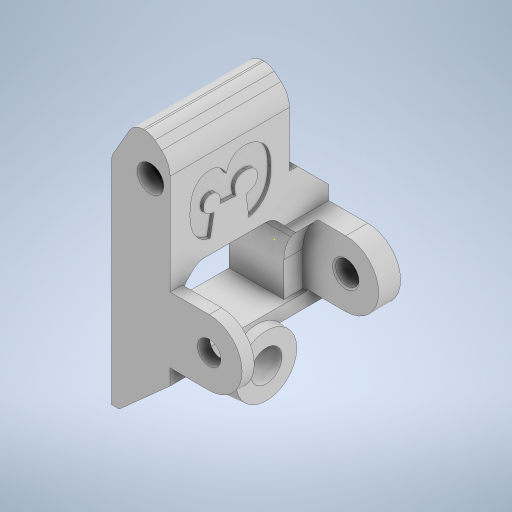
# Autodesk Inventor part: Extruder Idler V2
Saved by Autodesk Inventor 2023 (Build 270158000, 158)
## iProperties
Created: 2019-11-14
Part Number: Extruder Idler V2
Material: Generic
Document SubType Name: Modeling
Designer: pepd9
Density: 1 g/cm^3
Appearance: Default
Author: pepd9
Autodesk Inventor part; units mm, degrees
ref_plane "YZ Plane" through (0, 0, 0) normal (1, 0, 0) x (0, 1, 0)
ref_plane "XZ Plane" through (0, 0, 0) normal (0, 1, 0) x (-1, 0, 0)
ref_plane "XY Plane" through (0, 0, 0) normal (0, 0, 1) x (1, 0, 0)
sketch "Sketch1" plane through (0, 0, 0) normal (0, 0, 1) x (1, 0, 0)
  line L0 (-8.35, 16.25) -> (8.35, 16.25)
  line L1 (8.35, 16.25) -> (8.35, -16.25)
  line L2 (8.35, -16.25) -> (-8.35, -16.25)
  line L3 (-8.35, -16.25) -> (-8.35, 16.25)
  point P0 (0, 0)
  dimension "d2" = 16.7
  dimension "d3" = 8.35
  dimension "d4" = 32.5
  dimension "d5" = 16.25
  constraints: 8 end point, 2 parallel, 1 horizontal, 1 perpendicular
  measures "d2" distance of L0.start L0.end
  measures "d3" distance from line of L1 point (0, 0)
  measures "d4" distance of L0.end L1.end
  measures "d5" distance from line of point (0, 0) L0
extrude "Extrusion1" add sketch "Sketch1" along normal blind 25.5
sketch "Sketch3" plane through (0, 0, 0) normal (0, 0, -1) x (-1, 0, 0)
  line L0 (8.35, -16.25) -> (-8.35, -16.25) projected
  line L1 (8.35, 16.25) -> (8.35, -16.25) projected
  point P0 (0, 0)
  point P1 (-4.15, -4.25)
  dimension "d15" = 12
  dimension "d16" = 12.5
  measures "d15" distance from line of L0 point (-4.15, -4.25)
  measures "d16" distance from line of L1 point (-4.15, -4.25)
hole "Hole2" at (4.15, -4.25, 0) direction (0, 0, 1) diameter 2.99 end through all
sketch "Sketch4" plane through (0, 0, 0) normal (0, 0, -1) x (-1, 0, 0)
  line L0 (8.35, -16.25) -> (-8.35, -16.25) projected
  line L1 (-8.35, -16.25) -> (-8.35, 16.25) projected
  line L2 (8.35, 16.25) -> (8.35, -16.25) projected
  point P0 (0, 0)
  point P1 (3.35, 11.25)
  dimension "d24" = 27.5
  dimension "d36" = 5
  measures "d24" distance from line of L0 point (3.35, 11.25)
  measures "d36" distance from line of L2 point (3.35, 11.25)
hole "Hole3" at (-3.35, 11.25, 0) direction (0, 0, 1) diameter 3.4 end through all
sketch "Sketch5" plane through (0, 0, 0) normal (0, 0, -1) x (-1, 0, 0)
  circle A0 centre (3.35, 11.25) radius 1.7 projected
  line L0 (-8.35, 16.25) -> (8.35, 16.25) projected
  line L1 (8.35, 16.25) -> (8.35, -16.25) projected
  line L2 (-8.35, 16.25) -> (8.35, 16.25)
  line L3 (8.35, 16.25) -> (8.35, 5.75)
  line L4 (8.35, 5.75) -> (-8.35, 5.75)
  line L5 (-8.35, 5.75) -> (-8.35, 16.25)
  point P0 (0, 0)
  dimension "d33" = 5.5
  constraints: 8 end point, 2 parallel, 1 horizontal, 1 perpendicular, 1 point on line
  measures "d33" distance from line of L4 A0.centre
extrude "Extrusion2" cut sketch "Sketch5" against normal blind 5
sketch "Sketch6" plane through (0, 0, 0) normal (0, 0, -1) x (-1, 0, 0)
  line L0 (8.35, 5.75) -> (-8.35, 5.75) projected
  line L1 (-8.35, -16.25) -> (-8.35, 5.75) projected
  line L2 (8.35, -16.25) -> (-8.35, -16.25) projected
  line L3 (8.35, 5.75) -> (8.35, -16.25) projected
  circle A0 centre (-4.15, -4.25) radius 1.495 projected
  circle A1 centre (-4.15, -4.25) radius 4.2
  line L4 (-8.35, -16.25) -> (-8.35, 5.75) projected
  line L5 (-8.35, 5.75) -> (-8.35, 16.25) projected
  line L6 (8.35, 5.75) -> (-8.35, 5.75) projected
  line L7 (8.35, 16.25) -> (8.35, 5.75) projected
  line L8 (-8.35, 16.25) -> (8.35, 16.25) projected
  circle A2 centre (3.35, 11.25) radius 1.7 projected
  line L9 (-4.15, -0.05) -> (-2.65, -0.05)
  line L10 (-2.65, -0.05) -> (-2.65, 0.45)
  line L11 (-2.65, 0.45) -> (0.35, 16.25)
  line L12 (-8.35, 16.25) -> (8.35, 16.25) projected
  point P0 (0, 0)
  point P1 (0.35, 16.25)
  point P2 (-8.35, -4.25)
  dimension "d37" = 1.5
  dimension "d38" = 0.5
  dimension "d39" = 3
  constraints: 6 end point, 2 horizontal, 2 vertical, 1 coincident, 1 point on line, 3 other
  measures "d37" distance of L9.end L9.start
  measures "d38" distance of L9.end L10.end
  measures "d39" horizontal distance of A2.centre L11.end
extrude "Extrusion3" cut sketch "Sketch6" against normal through all contours L11 L10 L9 A1 L1 L0 | L0 L5 L8 L11
chamfer "Chamfer1" distance 3 angle 45 1 edges at (-0.35, 16.25, 15.25)
chamfer "Chamfer2" distance 5 angle 30 1 edges at (-8.35, 16.25, 15.25) measured on face at (-8.35, 15.75, 15.25)
ref_plane "Work Plane1" through (0, 0, 3.8) normal (0, 0, -1) x (-1, 0, 0)
sketch "Sketch7" plane through (0, 0, 3.8) normal (0, 0, -1) x (-1, 0, 0)
  arc A0 (-4.15, -0.05) -> (-8.35, -4.25) centre (-4.15, -4.25) ccw projected
  line L0 (-8.35, -16.25) -> (-8.35, -4.25) projected
  line L1 (8.35, -16.25) -> (-8.35, -16.25) projected
  line L2 (8.35, 5.75) -> (8.35, -16.25) projected
  line L3 (8.35, 5.75) -> (-1.6437, 5.75) projected
  line L4 (-1.6437, 5.75) -> (-2.65, 0.45) projected
  line L5 (-2.65, 0.45) -> (-2.65, -0.05) projected
  line L6 (-2.65, -0.05) -> (-4.15, -0.05) projected
  circle A1 centre (-4.15, -4.25) radius 1.495 projected
  circle A2 centre (-4.15, -4.25) radius 1.495 projected
  circle A3 centre (-4.15, -4.25) radius 5.5
  line L7 (1.35, -4.25) -> (-4.15, -4.25)
  line L8 (-4.15, -4.25) -> (-4.15, -9.75)
  line L9 (-4.15, -9.75) -> (1.35, -9.75)
  line L10 (1.35, -9.75) -> (1.35, -4.25)
  point P0 (0, 0)
  dimension "d49" = 11
  constraints: 8 end point, 2 parallel, 2 point on circle, 1 centre point, 1 coincident, 1 horizontal, 1 perpendicular
  measures "d49" diameter of A3
extrude "Extrusion4" cut sketch "Sketch7" against normal blind 5 contours L6 L5 L4 A3 L7 A1 L8 L0 A0 | A0 L0 A3 L4 L5 L6 | L8 A1 L7 A3 | A3 L10 L9 | L8 L7 A1 | A1 L7 L8
sketch "Sketch8" plane through (0, 0, 8.8) normal (0, 0, -1) x (-1, 0, 0)
  point P0 (0, 0)
sketch "Sketch9" plane through (0, 0, 8.8) normal (0, 0, -1) x (-1, 0, 0)
  circle A0 centre (-4.15, -4.25) radius 1.495 projected
  circle A1 centre (-4.15, -4.25) radius 5
  line L0 (-2.65, 0.45) -> (-2.5436, 1.0102) projected
  line L1 (-2.65, -0.05) -> (-2.65, 0.45) projected
  line L2 (-4.15, -0.05) -> (-2.65, -0.05) projected
  arc A2 (-4.15, -0.05) -> (-8.35, -4.25) centre (-4.15, -4.25) ccw projected
  line L3 (-8.35, -7.8011) -> (-8.35, -4.25) projected
  arc A3 (-8.35, -7.8011) -> (-4.15, -9.75) centre (-4.15, -4.25) ccw projected
  line L4 (1.35, -9.75) -> (-4.15, -9.75) projected
  line L5 (1.35, -4.25) -> (1.35, -9.75) projected
  arc A4 (1.35, -4.25) -> (-2.5436, 1.0102) centre (-4.15, -4.25) ccw projected
  circle A5 centre (-4.15, -4.25) radius 1.495 projected
  line L6 (-4.15, -9.25) -> (-9.15, -9.25)
  line L7 (-9.15, -9.25) -> (-9.15, -4.25)
  line L8 (-9.15, -4.25) -> (-4.15, -4.25)
  line L9 (-4.15, -4.25) -> (-4.15, -9.25)
  point P0 (0, 0)
  dimension "d52" = 10
  constraints: 8 end point, 2 parallel, 2 point on circle, 1 centre point, 1 coincident, 1 horizontal, 1 perpendicular
  measures "d52" diameter of A1
extrude "Extrusion5" cut sketch "Sketch9" against normal blind 9.4 contours A0 L8 A2 L2 L1 L0 A1 L9 | A0 L9 A1 L3 L8 | L8 A1 L0 L1 L2 A2 | L3 A1 L8 | L6 A3 L3 A1 | L3 A3 L6 L7 A1
ref_plane "Work Plane2" through (0, 0, 22) normal (0, 0, -1) x (-1, 0, 0)
sketch "Sketch10" plane through (0, 0, 22) normal (0, 0, -1) x (-1, 0, 0)
  circle A0 centre (-4.15, -4.25) radius 1.495 projected
  line L0 (-8.35, -9.25) -> (-8.35, -4.25) projected
  arc A1 (-4.15, -9.25) -> (-2.6375, 0.5158) centre (-4.15, -4.25) ccw projected
  line L1 (-2.65, 0.45) -> (-2.6375, 0.5158) projected
  line L2 (-2.65, -0.05) -> (-2.65, 0.45) projected
  line L3 (-4.15, -0.05) -> (-2.65, -0.05) projected
  arc A2 (-4.15, -0.05) -> (-8.35, -4.25) centre (-4.15, -4.25) ccw projected
  line L4 (-4.15, -9.25) -> (-8.35, -9.25) projected
  point P0 (0, 0)
extrude "Extrusion6" cut sketch "Sketch10" against normal through all
sketch "Sketch11" plane through (0, 0, 0) normal (0, 0, -1) x (-1, 0, 0)
  circle A0 centre (-4.15, -4.25) radius 1.495 projected
  line L0 (-1.6437, 5.75) -> (-2.65, 0.45) projected
  line L1 (-2.65, 0.45) -> (-2.65, -0.05) projected
  line L2 (-2.65, -0.05) -> (-4.15, -0.05) projected
  arc A1 (-4.15, -0.05) -> (-8.35, -4.25) centre (-4.15, -4.25) ccw projected
  line L3 (-8.35, -16.25) -> (-8.35, -4.25) projected
  line L4 (8.35, -16.25) -> (-8.35, -16.25) projected
  line L5 (8.35, 5.75) -> (8.35, -16.25) projected
  line L6 (8.35, 5.75) -> (-1.6437, 5.75) projected
  arc A2 (-4.15, -0.05) -> (-8.35, -4.25) centre (-4.15, -4.25) ccw projected
  circle A3 centre (-4.15, -4.25) radius 4.2
  line L7 (-4.15, -8.45) -> (0.85, -8.45)
  line L8 (8.35, -16.25) -> (-8.35, -16.25) projected
  line L9 (8.35, -16.25) -> (7.35, -16.25)
  line L10 (0.85, -8.45) -> (0.85, -10.45)
  line L11 (0.85, -10.45) -> (7.35, -16.25)
  point P0 (0, 0)
  dimension "d58" = 1
  dimension "d59" = 5
  dimension "d60" = 2
  constraints: 8 end point, 2 point on circle, 1 centre point, 1 coincident, 1 collinear, 1 horizontal, 1 point on line, 1 vertical
  measures "d58" distance of L4.start L9.end
  measures "d59" distance of L7.start L7.end
  measures "d60" distance of L7.end L10.end
extrude "Extrusion7" cut sketch "Sketch11" against normal through all contours L4 L3 A3 L7 L10 L11
fillet "Fillet1" radius 2 1 edges at (1.4371, -8.45, 23.75)
chamfer "Chamfer3" distance 0.2 angle 45 4 edges at (4.15, -5.745, 0) (4.15, -5.745, 18.2) (4.15, -5.745, 3.8) (4.15, -5.745, 22)
fillet "Fillet3" radius 2 4 edges at (0.2096, 13.3027, 15.25) (-3.35, 16.25, 15.25) (-5.4632, 16.25, 15.25) (-8.35, 11.25, 15.25)
sketch "Sketch12" plane through (-8.35, 5.75, 0) normal (-1, 0, 0) x (0, 0, 1)
  line L0 (18.1, -6.1) -> (18.1, -13.9) projected
  line L1 (3.8, -11.695) -> (3.8, -8.305) projected
  line L2 (3.8, -5.3) -> (3.8, -5.8) projected
  line L3 (3.8, -4.7398) -> (3.8, -5.3) projected
  line L4 (3.8, -10) -> (3.8, -4.7398) projected
  line L5 (3.8, -15.5) -> (3.8, -10) projected
  line L6 (18.2, -14.2) -> (18.2, -5.2342) projected
  line L7 (18.2, -14.2) -> (6.2, -14.2)
  line L8 (6.2, -14.2) -> (6.2, -4.2)
  line L9 (6.2, -4.2) -> (18.2, -4.2)
  line L10 (18.2, -4.2) -> (18.2, -14.2)
  line L11 (6.2, -14.2) -> (18.2, -14.2)
  line L12 (18.2, -14.2) -> (18.2, -16.2)
  line L13 (18.2, -16.2) -> (6.2, -16.2)
  line L14 (6.2, -16.2) -> (6.2, -14.2)
  line L15 (3.8, -15.5) -> (3.8, -14.2) projected
  line L16 (3.8, -14.2) -> (3.8, -5.8) projected
  point P0 (0, -5.75)
  dimension "d88" = 12
  dimension "d89" = 10
  dimension "d90" = 2
  constraints: 16 end point, 4 parallel, 2 horizontal, 2 perpendicular, 1 vertical alignment
  measures "d88" distance of L8.end L9.end
  measures "d89" distance of L7.end L8.end
  measures "d90" distance of L11.end L12.end
extrude "Extrusion8" cut sketch "Sketch12" against normal through all
sketch "Sketch13" plane through (-8.35, 5.75, 0) normal (-1, 0, 0) x (0, 0, 1)
  line L0 (5, 9.5) -> (5, 5.9641) projected
  line L1 (25.5, 5.9641) -> (25.5, 9.5) projected
  circle A0 centre (15.4, 10.3352) radius 2
  line L2 (15.4, 10.3352) -> (15.4, -24.7927)
  circle A1 centre (10.1533, -18.9) radius 4.5
  line L3 (18.1, -13.9) -> (5.8, -13.9) projected
  point P0 (0, -5.75)
  dimension "d81" = 4
  dimension "d82" = 9
  dimension "d83" = 5
  constraints: 2 centre point, 2 coincident, 2 end point, 1 vertical, 1 other
  measures "d81" diameter of A0
  measures "d82" diameter of A1
  measures "d83" distance from line of L3 point (10.153, -18.9)
extrude "Extrusion9" add sketch "Sketch13" against normal blind 8.7 contours A1
chamfer "Chamfer5" distance 2 angle 45 2 edges at (-2.9544, 1.55, 6.2) (-2.9544, 1.55, 18.2)
sketch "Sketch14" plane through (-8.35, 5.75, 0) normal (-1, 0, 0) x (0, 0, 1)
  arc A0 (6.8914, -22) -> (13.4152, -22) centre (10.1533, -18.9) ccw projected
  point P0 (0, -5.75)
hole "Hole4" at (-8.35, -13.15, 10.1533) direction (1, 0, 0) diameter 4 end through all counterbore diameter 7.4 counterbore depth 5
fillet "Fillet4" radius 2 2 edges at (-7.85, -16.25, 13.4152) (-7.85, -16.25, 6.8914)
fillet "Fillet5" radius 2 4 edges at (-1.2056, -0.45, 18.2) (-2.9544, 1.55, 16.2) (-2.9544, 1.55, 8.2) (-4.0881, -0.45, 6.2)
sketch "Sketch15" plane through (-8.35, -10.45, 6.2) normal (0, 0, 1) x (1, 0, 0)
  line L0 (0, 9.1716) -> (7.8719, 9.1716) projected
  line L1 (0, 0) -> (0, 9.1716) projected
  line L2 (0, 0) -> (7.5, 0) projected
  line L3 (7.5, 0.7) -> (7.5, 0) projected
  line L4 (7, 0.7) -> (7.5, 0.7) projected
  line L5 (7, 6.2) -> (7, 0.7) projected
  arc A0 (7.8719, 9.1716) -> (7, 6.2) centre (12.5, 6.2) ccw projected
  line L6 (0, 1.8) -> (8.7, 1.8) projected
  point P0 (8.35, 10.45)
  point P1 (7, 1.8)
extrude "Extrusion10" add sketch "Sketch15" along normal up to surface contours L6 L5 L4 L3 L2 L1 round surface about axis through (-8.35, -13.15, 10.1533) along (1, 0, 0) radius 4.5 far side no
sketch "Sketch16" plane through (0, 0, 18.2) normal (0, 0, -1) x (-1, 0, 0)
  line L0 (8.35, -8.65) -> (1.35, -8.65) projected
  line L1 (-7.1181, -1.2784) -> (8.35, -1.2784) projected
  arc A0 (-7.1181, -1.2784) -> (-4.15, -8.45) centre (-4.15, -4.25) ccw projected
  line L2 (-4.15, -8.45) -> (0.85, -8.45) projected
  line L3 (0.85, -10.45) -> (0.85, -8.45) projected
  line L4 (8.35, -10.45) -> (0.85, -10.45) projected
  line L5 (8.35, -1.2784) -> (8.35, -10.45) projected
  circle A1 centre (-4.15, -4.25) radius 1.695 projected
  line L6 (1.35, -8.65) -> (0.85, -8.65)
  line L7 (0.85, -10.45) -> (0.85, -8.45) projected
  point P0 (0, 0)
  constraints: 2 end point, 1 perpendicular, 1 point on line
extrude "Extrusion11" add sketch "Sketch16" along normal up to surface contours L5 L4 L3 L6 L0 round surface about axis through (-8.35, -13.15, 10.1533) along (1, 0, 0) radius 4.5 far side no
sketch "Sketch17" plane through (0, 0, 3.8) normal (0, 0, 1) x (1, 0, 0)
  arc A0 (-8.0821, 11.7141) -> (-8.35, 10.7141) centre (-6.35, 10.7141) ccw projected
  line L0 (-8.35, 10.7141) -> (-8.35, -16.25) projected
  line L1 (-8.35, -16.25) -> (-7.35, -16.25) projected
  line L2 (-7.35, -16.25) -> (-0.85, -10.45) projected
  line L3 (-0.85, -10.45) -> (-0.85, -8.45) projected
  arc A1 (-0.85, -8.45) -> (-0.4353, -6.2436) centre (-2.2695, -7.0411) ccw projected
  arc A2 (2.6375, 0.5158) -> (-0.4353, -6.2436) centre (4.15, -4.25) ccw projected
  line L4 (2.6375, 0.5158) -> (0.344, 12.5948) projected
  arc A3 (0.344, 12.5948) -> (-0.3454, 13.7622) centre (-1.6209, 12.2217) ccw projected
  line L5 (-2.795, 15.7905) -> (-0.3454, 13.7622) projected
  arc A4 (-2.795, 15.7905) -> (-4.0705, 16.25) centre (-4.0705, 14.25) ccw projected
  line L6 (-4.0705, 16.25) -> (-4.3085, 16.25) projected
  arc A5 (-4.3085, 16.25) -> (-6.0406, 15.25) centre (-4.3085, 14.25) ccw projected
  line L7 (-8.0821, 11.7141) -> (-6.0406, 15.25) projected
  circle A6 centre (-3.35, 11.25) radius 1.7 projected
  line L8 (-0.85, -9.75) -> (-0.85, -8.45) projected
  line L9 (-0.85, -8.45) -> (4.15, -8.45) projected
  arc A7 (4.15, -8.45) -> (4.15, -0.05) centre (4.15, -4.25) ccw projected
  line L10 (2.65, -0.05) -> (4.15, -0.05) projected
  line L11 (2.65, 0.45) -> (2.65, -0.05) projected
  line L12 (2.5436, 1.0102) -> (2.65, 0.45) projected
  arc A8 (2.5436, 1.0102) -> (-1.35, -4.25) centre (4.15, -4.25) ccw projected
  line L13 (-1.35, -9.75) -> (-1.35, -4.25) projected
  line L14 (-0.85, -9.75) -> (-1.35, -9.75) projected
  circle A9 centre (4.15, -4.25) radius 1.695 projected
  line L15 (-0.85, -8.45) -> (-1.35, -8.45)
  line L16 (-0.85, -8.65) -> (-1.35, -8.65) projected
  point P0 (0, 0)
  constraints: 2 end point, 1 horizontal, 1 point on line
extrude "Extrusion12" add sketch "Sketch17" along normal up to surface contours L14 L13 L16 L3 round surface about axis through (-8.35, -13.15, 10.1533) along (1, 0, 0) radius 4.5 far side no
chamfer "Chamfer6" distance 7 angle 5 1 edges at (0.35, -13.15, 5.6533) measured on face at (-0.15, -13.15, 5.6533)
sketch "Sketch18" plane through (0, 0, 25.5) normal (0, 0, 1) x (1, 0, 0)
  arc A0 (-8.0821, 11.7141) -> (-8.35, 10.7141) centre (-6.35, 10.7141) ccw projected
  line L0 (-8.35, 10.7141) -> (-8.35, -16.25) projected
  line L1 (-8.35, -16.25) -> (-7.35, -16.25) projected
  line L2 (-7.35, -16.25) -> (-0.85, -10.45) projected
  line L3 (-0.85, -10.45) -> (-0.85, -8.45) projected
  arc A1 (-0.85, -8.45) -> (-0.4353, -6.2436) centre (-2.2695, -7.0411) ccw projected
  arc A2 (2.6375, 0.5158) -> (-0.4353, -6.2436) centre (4.15, -4.25) ccw projected
  line L4 (2.6375, 0.5158) -> (0.344, 12.5948) projected
  arc A3 (0.344, 12.5948) -> (-0.3454, 13.7622) centre (-1.6209, 12.2217) ccw projected
  line L5 (-2.795, 15.7905) -> (-0.3454, 13.7622) projected
  arc A4 (-2.795, 15.7905) -> (-4.0705, 16.25) centre (-4.0705, 14.25) ccw projected
  line L6 (-4.0705, 16.25) -> (-4.3085, 16.25) projected
  arc A5 (-4.3085, 16.25) -> (-6.0406, 15.25) centre (-4.3085, 14.25) ccw projected
  line L7 (-8.0821, 11.7141) -> (-6.0406, 15.25) projected
  circle A6 centre (-3.35, 11.25) radius 1.7 projected
  point P0 (0, 0)
extrude "Extrusion13" cut sketch "Sketch18" against normal up to surface (3.5 mm away)
move faces "Move1" translate (0, 0, 1.5) faces at (-2.2442, -4.5914, 18.2) (1.745, -0.9695, 18.176) (-1.0492, 0.4119, 17.3381) (-1.1002, 1.1525, 16.5682)
move faces "Move2" translate (0, 0, -0.75) faces at (-5.85, -4.662, 22)
move faces "Move3" translate (0, 0, 1) faces at (-5.85, -6.3167, 0)
move faces "Move4" translate (0, 0, 1) faces at (-3.3521, 7.0167, 5)
sketch "Sketch19" plane through (2.65, -0.05, 21.25) normal (1, 0, 0) x (0, 0, -1)
  line L0 (20.25, 5.8) -> (20.25, 0.5) projected
  line L1 (15.25, 16.3) -> (0, 16.3) projected
  line L2 (0, 0) -> (20.25, 0)
  line L3 (20.25, 0) -> (20.25, 16.3)
  line L4 (20.25, 16.3) -> (0, 16.3)
  line L5 (0, 16.3) -> (0, 0)
  point P0 (21.25, 0.05)
  point P1 (20.25, 0.5)
  constraints: 8 end point, 2 parallel, 1 horizontal, 1 perpendicular
extrude "Extrusion14" cut sketch "Sketch19" against normal blind 3.5
fillet "Fillet6" radius 3 1 edges at (-0.85, 14.18, 13.625)
sketch "Sketch20" plane through (-0.85, -0.05, 21.25) normal (1, 0, 0) x (0, 0, -1)
  line L0 (2.5245, 2.7393) -> (2.5245, 26.0502) construction
  line L1 (2.5245, 26.0502) -> (12.6977, 26.0502) construction
  line L2 (12.6977, 26.0502) -> (12.6977, 2.7393) construction
  line L3 (12.6977, 2.7393) -> (2.5245, 2.7393) construction
  line L4 (5.5851, 6.0117) -> (5.1135, 3.3842)
  spline S0 degree 2 poles (5.1135, 3.3842) (3.8623, 3.7114) (2.5245, 5.5689) (2.5245, 7.2725) knots 0 0 0 1 2 2 2
  spline S1 degree 2 poles (2.5245, 7.2725) (2.5245, 9.2359) (3.9874, 10.978) (5.0846, 10.978) knots 0 0 0 1 2 2 2
  spline S2 degree 2 poles (5.0846, 10.978) (5.7391, 10.978) (6.7882, 10.2658) (7.1828, 9.5439) knots 0 0 0 1 2 2 2
  spline S3 degree 2 poles (7.1828, 9.5439) (7.3272, 10.131) (7.5197, 10.439) knots 0 0 0 1 1 1
  spline S4 degree 2 poles (7.5197, 10.439) (7.8276, 10.9395) (8.8286, 11.4881) (9.5216, 11.4881) knots 0 0 0 1 2 2 2
  spline S5 degree 2 poles (9.5216, 11.4881) (10.3974, 11.4881) (12.0047, 10.5738) (12.8709, 8.8606) (12.8709, 7.4554) knots 0 0 0 1 2 3 3 3
  spline S6 degree 2 poles (12.8709, 7.4554) (12.8709, 6.0983) (12.2261, 4.5199) (10.9941, 3.4997) (10.0606, 3.2302) knots 0 0 0 1 2 3 3 3
  line L5 (10.0606, 3.2302) -> (9.6948, 6.0117)
  spline S7 degree 2 poles (9.6948, 6.0117) (10.5322, 6.1753) (11.177, 6.8586) (11.177, 7.388) knots 0 0 0 1 2 2 2
  spline S8 degree 2 poles (11.177, 7.388) (11.177, 7.9462) (10.3589, 8.6873) (9.6756, 8.6873) knots 0 0 0 1 2 2 2
  spline S9 degree 2 poles (9.6756, 8.6873) (8.973, 8.6873) (8.2126, 7.9751) (8.2126, 7.3591) knots 0 0 0 1 2 2 2
  spline S10 degree 2 poles (8.2126, 7.3591) (8.2126, 7.0319) (8.3762, 6.464) knots 0 0 0 1 1 1
  line L6 (8.3762, 6.464) -> (6.3839, 6.6084)
  spline S11 degree 2 poles (6.3839, 6.6084) (6.4224, 6.8394) (6.4224, 6.9645) knots 0 0 0 1 1 1
  spline S12 degree 2 poles (6.4224, 6.9645) (6.4224, 7.5131) (5.7295, 8.2446) (5.2482, 8.2446) knots 0 0 0 1 2 2 2
  spline S13 degree 2 poles (5.2482, 8.2446) (4.7959, 8.2446) (4.2473, 7.696) (4.2473, 7.2244) knots 0 0 0 1 2 2 2
  spline S14 degree 2 poles (4.2473, 7.2244) (4.2473, 6.7335) (4.844, 6.1176) (5.5851, 6.0117) knots 0 0 0 1 2 2 2
  point P0 (21.25, 0.05)
  constraints: 2 other
extrude "Extrusion15" cut sketch "Sketch20" against normal blind 0.4
chamfer "Chamfer7" distance 4 angle 45 1 edges at (-4.6, 5.75, 1)
sketch "Sketch21" plane through (-0.85, -0.05, 21.25) normal (1, 0, 0) x (0, 0, -1)
  line L0 (16.25, 5.8) -> (20.25, 1.8) projected
  line L1 (15.25, 5.8) -> (16.25, 5.8) projected
  line L2 (15.25, 12.8191) -> (15.25, 5.8) projected
  line L3 (0, 12.8191) -> (15.25, 12.8191) projected
  line L4 (0, 0) -> (0, 12.8191) projected
  line L5 (1.9717, 0) -> (0, 0) projected
  arc A0 (2.1358, 0.1858) -> (1.9717, 0) centre (3.55, -1.2284) ccw projected
  line L6 (2.9642, 1.0142) -> (2.1358, 0.1858) projected
  arc A1 (4.3784, 1.6) -> (2.9642, 1.0142) centre (4.3784, -0.4) ccw projected
  line L7 (12.2216, 1.6) -> (4.3784, 1.6) projected
  arc A2 (13.6358, 1.0142) -> (12.2216, 1.6) centre (12.2216, -0.4) ccw projected
  line L8 (14.4642, 0.1858) -> (13.6358, 1.0142) projected
  arc A3 (14.6283, 0) -> (14.4642, 0.1858) centre (13.05, -1.2284) ccw projected
  line L9 (20.25, 0) -> (14.6283, 0) projected
  line L10 (20.25, 1.8) -> (20.25, 0) projected
  line L11 (5.5851, 6.0117) -> (5.1135, 3.3842) projected
  line L12 (10.0606, 3.2302) -> (9.6948, 6.0117) projected
  line L13 (8.3762, 6.464) -> (6.3839, 6.6084) projected
  line L14 (0, -8.4) -> (0, 0) projected
  line L15 (1.55, -8.4) -> (0, -8.4) projected
  line L16 (1.55, -8.4) -> (1.55, -1.2284) projected
  line L17 (1.9717, 0) -> (0, 0) projected
  arc A4 (2.1358, 0.1858) -> (1.55, -1.2284) centre (3.55, -1.2284) ccw projected
  line L18 (1.55, -1.2284) -> (2.1358, -1.2284)
  line L19 (2.1358, -1.2284) -> (2.1358, 0.1858)
  line L20 (2.1358, 0.1858) -> (1.55, 0.1858)
  line L21 (1.55, 0.1858) -> (1.55, -1.2284)
  point P0 (21.25, 0.05)
  constraints: 8 end point, 2 parallel, 1 horizontal, 1 perpendicular, 16 other
extrude "Extrusion16" cut sketch "Sketch21" along normal through all contours L21 L20 A0 L5 | L5 A4 L21 | A0 L19 L18 A4
body "Solid1"
